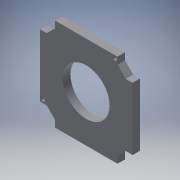
# Autodesk Inventor part: 20_Cube_Insert_CirAp_Guide
Saved by Autodesk Inventor 2019 (Build 230136000, 136)
## iProperties
Created: 2019-10-23
Part Number: 20_Cube_Insert_CirAp_Guide
Material: Generic
Document SubType Name: Modeling
Designer: marsikovabarbora
Density: 1 g/cm^3
Appearance: Default
Author: marsikovabarbora
Autodesk Inventor part; units mm, degrees
ref_plane "YZ Plane" through (0, 0, 0) normal (1, 0, 0) x (0, 1, 0)
ref_plane "XZ Plane" through (0, 0, 0) normal (0, 1, 0) x (-1, 0, 0)
ref_plane "XY Plane" through (0, 0, 0) normal (0, 0, 1) x (1, 0, 0)
sketch "Sketch1" plane through (0, 0, 0) normal (0, 0, 1) x (1, 0, 0)
  line L0 (-34.8609, 0) -> (34.8609, 0) construction
  line L1 (0, -34.8609) -> (0, 34.8609) construction
  line L2 (0, 0) -> (11.6542, 11.6542) construction
  line L3 (0, 0) -> (16.4815, 0) construction
  line L4 (0, 24.9006) -> (16.8, 24.9006)
  line L5 (16.8, 24.9006) -> (16.8, 21.2406)
  line L6 (16.8, 21.2406) -> (19.0203, 19.0203)
  line L7 (24.9006, 0) -> (24.9006, 16.8)
  line L8 (24.9006, 16.8) -> (21.2406, 16.8)
  line L9 (21.2406, 16.8) -> (19.0203, 19.0203)
  line L10 (0, 0) -> (-11.6542, 11.6542) construction
  line L11 (0, 0) -> (-16.4815, 0) construction
  line L12 (0, 24.9006) -> (-16.8, 24.9006)
  line L13 (-16.8, 24.9006) -> (-16.8, 21.2406)
  line L14 (-16.8, 21.2406) -> (-19.0203, 19.0203)
  line L15 (-24.9006, 0) -> (-24.9006, 16.8)
  line L16 (-24.9006, 16.8) -> (-21.2406, 16.8)
  line L17 (-21.2406, 16.8) -> (-19.0203, 19.0203)
  line L18 (0, 0) -> (11.6542, -11.6542) construction
  line L19 (0, -24.9006) -> (16.8, -24.9006)
  line L20 (16.8, -24.9006) -> (16.8, -21.2406)
  line L21 (16.8, -21.2406) -> (19.0203, -19.0203)
  line L22 (24.9006, 0) -> (24.9006, -16.8)
  line L23 (24.9006, -16.8) -> (21.2406, -16.8)
  line L24 (21.2406, -16.8) -> (19.0203, -19.0203)
  line L25 (0, 0) -> (-11.6542, -11.6542) construction
  line L26 (0, -24.9006) -> (-16.8, -24.9006)
  line L27 (-16.8, -24.9006) -> (-16.8, -21.2406)
  line L28 (-16.8, -21.2406) -> (-19.0203, -19.0203)
  line L29 (-24.9006, 0) -> (-24.9006, -16.8)
  line L30 (-24.9006, -16.8) -> (-21.2406, -16.8)
  line L31 (-21.2406, -16.8) -> (-19.0203, -19.0203)
  dimension "d0" = 45
  dimension "d1" = 3.14
  dimension "d2" = 3.66
  dimension "d3" = 16.8
  constraints: 60 end point, 24 symmetric about line, 5 point on line, 2 horizontal, 2 perpendicular, 1 equal length
  measures "d0" angle of L3 L2
  measures "d1" distance of L5.end L6.end
  measures "d2" distance of L4.end L5.end
  measures "d3" distance of L4.start L4.end
extrude "Extrusion1" add sketch "Sketch1" along normal blind 4
hole "Hole1" at (0, 0, 0) direction (0, 0, 1) diameter 26.6 end through all
sketch "Sketch6" plane through (0, 0, 4) normal (0, 0, 1) x (1, 0, 0)
  circle A0 centre (0, 0) radius 13.3 construction
  line L0 (16.8, 24.9006) -> (-16.8, 24.9006) construction
  line L1 (-16.8, 24.9006) -> (-16.8, 21.2406) construction
  line L2 (-16.8, 21.2406) -> (-21.2406, 16.8) construction
  line L3 (-21.2406, 16.8) -> (-24.9006, 16.8) construction
  line L4 (-24.9006, 16.8) -> (-24.9006, -16.8) construction
  line L5 (-24.9006, -16.8) -> (-21.2406, -16.8) construction
  line L6 (-21.2406, -16.8) -> (-16.8, -21.2406) construction
  line L7 (-16.8, -21.2406) -> (-16.8, -24.9006) construction
  line L8 (-16.8, -24.9006) -> (16.8, -24.9006) construction
  line L9 (16.8, -24.9006) -> (16.8, -21.2406) construction
  line L10 (16.8, -21.2406) -> (21.2406, -16.8) construction
  line L11 (21.2406, -16.8) -> (24.9006, -16.8) construction
  line L12 (24.9006, -16.8) -> (24.9006, 16.8) construction
  line L13 (24.9006, 16.8) -> (21.2406, 16.8) construction
  line L14 (21.2406, 16.8) -> (16.8, 21.2406) construction
  line L15 (16.8, 21.2406) -> (16.8, 24.9006) construction
  circle A1 centre (0, 0) radius 13.3
  circle A2 centre (0, 0) radius 13.5
  dimension "d42" = 26.6
  dimension "d43" = 27
  constraints: 2 centre point, 1 coincident, 1 concentric
  measures "d42" diameter of A1
  measures "d43" diameter of A2
extrude "Extrusion4" [suppressed]
sketch "Sketch7" plane through (0, 0, 0) normal (0, 0, -1) x (-1, 0, 0)
  line L0 (16.8, 24.9006) -> (-16.8, 24.9006) construction
  line L1 (-16.8, 24.9006) -> (-16.8, 21.2406) construction
  line L2 (-16.8, 21.2406) -> (-21.2406, 16.8) construction
  line L3 (-21.2406, 16.8) -> (-24.9006, 16.8) construction
  line L4 (-24.9006, 16.8) -> (-24.9006, -16.8) construction
  line L5 (-24.9006, -16.8) -> (-21.2406, -16.8) construction
  line L6 (-21.2406, -16.8) -> (-16.8, -21.2406) construction
  line L7 (-16.8, -21.2406) -> (-16.8, -24.9006) construction
  line L8 (-16.8, -24.9006) -> (16.8, -24.9006) construction
  line L9 (16.8, -24.9006) -> (16.8, -21.2406) construction
  line L10 (16.8, -21.2406) -> (21.2406, -16.8) construction
  line L11 (21.2406, -16.8) -> (24.9006, -16.8) construction
  line L12 (24.9006, -16.8) -> (24.9006, 16.8) construction
  line L13 (24.9006, 16.8) -> (21.2406, 16.8) construction
  line L14 (21.2406, 16.8) -> (16.8, 21.2406) construction
  line L15 (16.8, 21.2406) -> (16.8, 24.9006) construction
  line L16 (-2.0147, 24.1761) -> (-2, 24) construction
  line L17 (-1.9775, 24.0019) -> (-1.9921, 24.178) construction
  line L18 (1.9921, 24.178) -> (1.9775, 24.0019) construction
  line L19 (2, 24) -> (2.0147, 24.1761) construction
  line L20 (5.9445, 23.5204) -> (5.9012, 23.349) construction
  line L21 (5.923, 23.3435) -> (5.9665, 23.5148) construction
  line L22 (9.7347, 22.2212) -> (9.6638, 22.0593) construction
  line L23 (9.6844, 22.0502) -> (9.7555, 22.212) construction
  line L24 (13.2594, 20.3158) -> (13.1628, 20.1678) construction
  line L25 (13.1817, 20.1555) -> (13.2784, 20.3034) construction
  line L26 (16.4225, 17.8563) -> (16.3028, 17.7262) construction
  line L27 (16.3194, 17.7109) -> (16.4392, 17.8409) construction
  line L28 (19.1375, 14.9097) -> (18.9981, 14.8011) construction
  line L29 (19.0119, 14.7833) -> (19.1515, 14.8918) construction
  line L30 (21.3306, 11.5564) -> (21.1752, 11.4722) construction
  line L31 (21.1859, 11.4524) -> (21.3414, 11.5365) construction
  line L32 (22.9418, 7.8879) -> (22.7746, 7.8305) construction
  line L33 (22.782, 7.8091) -> (22.9492, 7.8665) construction
  line L34 (23.9272, 4.0042) -> (23.7529, 3.9751) construction
  line L35 (23.7566, 3.9529) -> (23.9309, 3.9819) construction
  line L36 (24.2599, 0.0113) -> (24.0832, 0.0113) construction
  line L37 (24.0832, -0.0113) -> (24.2599, -0.0113) construction
  line L38 (23.9309, -3.9819) -> (23.7566, -3.9529) construction
  line L39 (23.7529, -3.9751) -> (23.9272, -4.0042) construction
  line L40 (22.9492, -7.8665) -> (22.782, -7.8091) construction
  line L41 (22.7746, -7.8305) -> (22.9418, -7.8879) construction
  line L42 (21.3414, -11.5365) -> (21.1859, -11.4524) construction
  line L43 (21.1752, -11.4722) -> (21.3306, -11.5564) construction
  line L44 (19.1515, -14.8918) -> (19.0119, -14.7833) construction
  line L45 (18.9981, -14.8011) -> (19.1375, -14.9097) construction
  line L46 (16.4392, -17.8409) -> (16.3194, -17.7109) construction
  line L47 (16.3028, -17.7262) -> (16.4225, -17.8563) construction
  line L48 (13.2784, -20.3034) -> (13.1817, -20.1555) construction
  line L49 (13.1628, -20.1678) -> (13.2594, -20.3158) construction
  line L50 (9.7555, -22.212) -> (9.6844, -22.0502) construction
  line L51 (9.6638, -22.0593) -> (9.7347, -22.2212) construction
  line L52 (5.9665, -23.5148) -> (5.923, -23.3435) construction
  line L53 (5.9012, -23.349) -> (5.9445, -23.5204) construction
  line L54 (2.0147, -24.1761) -> (2, -24) construction
  line L55 (1.9775, -24.0019) -> (1.9921, -24.178) construction
  line L56 (-1.9921, -24.178) -> (-1.9775, -24.0019) construction
  line L57 (-2, -24) -> (-2.0147, -24.1761) construction
  line L58 (-5.9445, -23.5204) -> (-5.9012, -23.349) construction
  line L59 (-5.923, -23.3435) -> (-5.9665, -23.5148) construction
  line L60 (-9.7347, -22.2212) -> (-9.6638, -22.0593) construction
  line L61 (-9.6844, -22.0502) -> (-9.7555, -22.212) construction
  line L62 (-13.2594, -20.3158) -> (-13.1628, -20.1678) construction
  line L63 (-13.1817, -20.1555) -> (-13.2784, -20.3034) construction
  line L64 (-16.4225, -17.8563) -> (-16.3028, -17.7262) construction
  line L65 (-16.3194, -17.7109) -> (-16.4392, -17.8409) construction
  line L66 (-19.1375, -14.9097) -> (-18.9981, -14.8011) construction
  line L67 (-19.0119, -14.7833) -> (-19.1515, -14.8918) construction
  line L68 (-21.3306, -11.5564) -> (-21.1752, -11.4722) construction
  line L69 (-21.1859, -11.4524) -> (-21.3414, -11.5365) construction
  line L70 (-22.9418, -7.8879) -> (-22.7746, -7.8305) construction
  line L71 (-22.782, -7.8091) -> (-22.9492, -7.8665) construction
  line L72 (-23.9272, -4.0042) -> (-23.7529, -3.9751) construction
  line L73 (-23.7566, -3.9529) -> (-23.9309, -3.9819) construction
  line L74 (-24.2599, -0.0113) -> (-24.0832, -0.0113) construction
  line L75 (-24.0832, 0.0113) -> (-24.2599, 0.0113) construction
  line L76 (-23.9309, 3.9819) -> (-23.7566, 3.9529) construction
  line L77 (-23.7529, 3.9751) -> (-23.9272, 4.0042) construction
  line L78 (-22.9492, 7.8665) -> (-22.782, 7.8091) construction
  line L79 (-22.7746, 7.8305) -> (-22.9418, 7.8879) construction
  line L80 (-21.3414, 11.5365) -> (-21.1859, 11.4524) construction
  line L81 (-21.1752, 11.4722) -> (-21.3306, 11.5564) construction
  line L82 (-19.1515, 14.8918) -> (-19.0119, 14.7833) construction
  line L83 (-18.9981, 14.8011) -> (-19.1375, 14.9097) construction
  line L84 (-16.4392, 17.8409) -> (-16.3194, 17.7109) construction
  line L85 (-16.3028, 17.7262) -> (-16.4225, 17.8563) construction
  line L86 (-13.2784, 20.3034) -> (-13.1817, 20.1555) construction
  line L87 (-13.1628, 20.1678) -> (-13.2594, 20.3158) construction
  line L88 (-9.7555, 22.212) -> (-9.6844, 22.0502) construction
  line L89 (-9.6638, 22.0593) -> (-9.7347, 22.2212) construction
  line L90 (-5.9665, 23.5148) -> (-5.923, 23.3435) construction
  line L91 (-5.9012, 23.349) -> (-5.9445, 23.5204) construction
  circle A0 centre (0, 24.5946) radius 2 construction
  line L92 (2, 33.2113) -> (-2, 33.2113)
  line L93 (-2, 33.2113) -> (-2, 6.8481)
  line L94 (-2, 6.8481) -> (2, 6.8481)
  line L95 (2, 6.8481) -> (2, 33.2113)
  circle A1 centre (-17.7867, 14.1844) radius 1.25 projected
  circle A2 centre (-22.1796, -5.0624) radius 1.25 projected
  circle A3 centre (-9.8709, -20.497) radius 1.25 projected
  circle A4 centre (9.8709, -20.497) radius 1.25 projected
  circle A5 centre (22.1796, -5.0624) radius 1.25 projected
  circle A6 centre (17.7867, 14.1844) radius 1.25 projected
  circle A7 centre (0, 22.75) radius 1.25 projected
  arc A8 (-2.0147, 24.1761) -> (-5.9445, 23.5204) centre (-3.9503, 23.6727) ccw projected
  arc A9 (-1.9973, 24.1039) -> (-2, 24) centre (0, 24) ccw projected
  arc A10 (-1.9775, 24.0019) -> (-1.9973, 24.1039) centre (-3.9503, 23.6727) ccw projected
  arc A11 (1.9921, 24.178) -> (-1.9921, 24.178) centre (0, 24) ccw projected
  arc A12 (1.9973, 24.1039) -> (1.9775, 24.0019) centre (3.9503, 23.6727) ccw projected
  arc A13 (2, 24) -> (1.9973, 24.1039) centre (0, 24) ccw projected
  arc A14 (5.9445, 23.5204) -> (2.0147, 24.1761) centre (3.9503, 23.6727) ccw projected
  arc A15 (5.9374, 23.4464) -> (5.9012, 23.349) centre (7.7928, 22.6996) ccw projected
  arc A16 (5.923, 23.3435) -> (5.9374, 23.4464) centre (3.9503, 23.6727) ccw projected
  arc A17 (9.7347, 22.2212) -> (5.9665, 23.5148) centre (7.7928, 22.6996) ccw projected
  arc A18 (9.7156, 22.1493) -> (9.6638, 22.0593) centre (11.4227, 21.1074) ccw projected
  arc A19 (9.6844, 22.0502) -> (9.7156, 22.1493) centre (7.7928, 22.6996) ccw projected
  arc A20 (13.2594, 20.3158) -> (9.7555, 22.212) centre (11.4227, 21.1074) ccw projected
  arc A21 (13.2287, 20.2481) -> (13.1628, 20.1678) centre (14.7411, 18.9394) ccw projected
  arc A22 (13.1817, 20.1555) -> (13.2287, 20.2481) centre (11.4227, 21.1074) ccw projected
  arc A23 (16.4225, 17.8563) -> (13.2784, 20.3034) centre (14.7411, 18.9394) ccw projected
  arc A24 (16.381, 17.7946) -> (16.3028, 17.7262) centre (17.6574, 16.2548) ccw projected
  arc A25 (16.3194, 17.7109) -> (16.381, 17.7946) centre (14.7411, 18.9394) ccw projected
  arc A26 (19.1375, 14.9097) -> (16.4392, 17.8409) centre (17.6574, 16.2548) ccw projected
  arc A27 (19.0865, 14.8556) -> (18.9981, 14.8011) centre (20.092, 13.1268) ccw projected
  arc A28 (19.0119, 14.7833) -> (19.0865, 14.8556) centre (17.6574, 16.2548) ccw projected
  arc A29 (21.3306, 11.5564) -> (19.1515, 14.8918) centre (20.092, 13.1268) ccw projected
  arc A30 (21.2714, 11.5115) -> (21.1752, 11.4722) centre (21.9786, 9.6407) ccw projected
  arc A31 (21.1859, 11.4524) -> (21.2714, 11.5115) centre (20.092, 13.1268) ccw projected
  arc A32 (22.9418, 7.8879) -> (21.3414, 11.5365) centre (21.9786, 9.6407) ccw projected
  arc A33 (22.876, 7.8533) -> (22.7746, 7.8305) centre (23.2656, 5.8917) ccw projected
  arc A34 (22.782, 7.8091) -> (22.876, 7.8533) centre (21.9786, 9.6407) ccw projected
  arc A35 (23.9272, 4.0042) -> (22.9492, 7.8665) centre (23.2656, 5.8917) ccw projected
  arc A36 (23.8566, 3.981) -> (23.7529, 3.9751) centre (23.918, 1.9819) ccw projected
  arc A37 (23.7566, 3.9529) -> (23.8566, 3.981) centre (23.2656, 5.8917) ccw projected
  arc A38 (24.2599, 0.0113) -> (23.9309, 3.9819) centre (23.918, 1.9819) ccw projected
  arc A39 (24.1865, 0) -> (24.0832, 0.0113) centre (23.918, -1.9819) ccw projected
  arc A40 (24.0832, -0.0113) -> (24.1865, 0) centre (23.918, 1.9819) ccw projected
  arc A41 (23.9309, -3.9819) -> (24.2599, -0.0113) centre (23.918, -1.9819) ccw projected
  arc A42 (23.8566, -3.981) -> (23.7566, -3.9529) centre (23.2656, -5.8917) ccw projected
  arc A43 (23.7529, -3.9751) -> (23.8566, -3.981) centre (23.918, -1.9819) ccw projected
  arc A44 (22.9492, -7.8665) -> (23.9272, -4.0042) centre (23.2656, -5.8917) ccw projected
  arc A45 (22.876, -7.8533) -> (22.782, -7.8091) centre (21.9786, -9.6407) ccw projected
  arc A46 (22.7746, -7.8305) -> (22.876, -7.8533) centre (23.2656, -5.8917) ccw projected
  arc A47 (21.3414, -11.5365) -> (22.9418, -7.8879) centre (21.9786, -9.6407) ccw projected
  arc A48 (21.2714, -11.5115) -> (21.1859, -11.4524) centre (20.092, -13.1268) ccw projected
  arc A49 (21.1752, -11.4722) -> (21.2714, -11.5115) centre (21.9786, -9.6407) ccw projected
  arc A50 (19.1515, -14.8918) -> (21.3306, -11.5564) centre (20.092, -13.1268) ccw projected
  arc A51 (19.0865, -14.8556) -> (19.0119, -14.7833) centre (17.6574, -16.2548) ccw projected
  arc A52 (18.9981, -14.8011) -> (19.0865, -14.8556) centre (20.092, -13.1268) ccw projected
  arc A53 (16.4392, -17.8409) -> (19.1375, -14.9097) centre (17.6574, -16.2548) ccw projected
  arc A54 (16.381, -17.7946) -> (16.3194, -17.7109) centre (14.7411, -18.9394) ccw projected
  arc A55 (16.3028, -17.7262) -> (16.381, -17.7946) centre (17.6574, -16.2548) ccw projected
  arc A56 (13.2784, -20.3034) -> (16.4225, -17.8563) centre (14.7411, -18.9394) ccw projected
  arc A57 (13.2287, -20.2481) -> (13.1817, -20.1555) centre (11.4227, -21.1074) ccw projected
  arc A58 (13.1628, -20.1678) -> (13.2287, -20.2481) centre (14.7411, -18.9394) ccw projected
  arc A59 (9.7555, -22.212) -> (13.2594, -20.3158) centre (11.4227, -21.1074) ccw projected
  arc A60 (9.7156, -22.1493) -> (9.6844, -22.0502) centre (7.7928, -22.6996) ccw projected
  arc A61 (9.6638, -22.0593) -> (9.7156, -22.1493) centre (11.4227, -21.1074) ccw projected
  arc A62 (5.9665, -23.5148) -> (9.7347, -22.2212) centre (7.7928, -22.6996) ccw projected
  arc A63 (5.9374, -23.4464) -> (5.923, -23.3435) centre (3.9503, -23.6727) ccw projected
  arc A64 (5.9012, -23.349) -> (5.9374, -23.4464) centre (7.7928, -22.6996) ccw projected
  arc A65 (2.0147, -24.1761) -> (5.9445, -23.5204) centre (3.9503, -23.6727) ccw projected
  arc A66 (1.9973, -24.1039) -> (2, -24) centre (0, -24) ccw projected
  arc A67 (1.9775, -24.0019) -> (1.9973, -24.1039) centre (3.9503, -23.6727) ccw projected
  arc A68 (-1.9921, -24.178) -> (1.9921, -24.178) centre (0, -24) ccw projected
  arc A69 (-1.9973, -24.1039) -> (-1.9775, -24.0019) centre (-3.9503, -23.6727) ccw projected
  arc A70 (-2, -24) -> (-1.9973, -24.1039) centre (0, -24) ccw projected
  arc A71 (-5.9445, -23.5204) -> (-2.0147, -24.1761) centre (-3.9503, -23.6727) ccw projected
  arc A72 (-5.9374, -23.4464) -> (-5.9012, -23.349) centre (-7.7928, -22.6996) ccw projected
  arc A73 (-5.923, -23.3435) -> (-5.9374, -23.4464) centre (-3.9503, -23.6727) ccw projected
  arc A74 (-9.7347, -22.2212) -> (-5.9665, -23.5148) centre (-7.7928, -22.6996) ccw projected
  arc A75 (-9.7156, -22.1493) -> (-9.6638, -22.0593) centre (-11.4227, -21.1074) ccw projected
  arc A76 (-9.6844, -22.0502) -> (-9.7156, -22.1493) centre (-7.7928, -22.6996) ccw projected
  arc A77 (-13.2594, -20.3158) -> (-9.7555, -22.212) centre (-11.4227, -21.1074) ccw projected
  arc A78 (-13.2287, -20.2481) -> (-13.1628, -20.1678) centre (-14.7411, -18.9394) ccw projected
  arc A79 (-13.1817, -20.1555) -> (-13.2287, -20.2481) centre (-11.4227, -21.1074) ccw projected
  arc A80 (-16.4225, -17.8563) -> (-13.2784, -20.3034) centre (-14.7411, -18.9394) ccw projected
  arc A81 (-16.381, -17.7946) -> (-16.3028, -17.7262) centre (-17.6574, -16.2548) ccw projected
  arc A82 (-16.3194, -17.7109) -> (-16.381, -17.7946) centre (-14.7411, -18.9394) ccw projected
  arc A83 (-19.1375, -14.9097) -> (-16.4392, -17.8409) centre (-17.6574, -16.2548) ccw projected
  arc A84 (-19.0865, -14.8556) -> (-18.9981, -14.8011) centre (-20.092, -13.1268) ccw projected
  arc A85 (-19.0119, -14.7833) -> (-19.0865, -14.8556) centre (-17.6574, -16.2548) ccw projected
  arc A86 (-21.3306, -11.5564) -> (-19.1515, -14.8918) centre (-20.092, -13.1268) ccw projected
  arc A87 (-21.2714, -11.5115) -> (-21.1752, -11.4722) centre (-21.9786, -9.6407) ccw projected
  arc A88 (-21.1859, -11.4524) -> (-21.2714, -11.5115) centre (-20.092, -13.1268) ccw projected
  arc A89 (-22.9418, -7.8879) -> (-21.3414, -11.5365) centre (-21.9786, -9.6407) ccw projected
  arc A90 (-22.876, -7.8533) -> (-22.7746, -7.8305) centre (-23.2656, -5.8917) ccw projected
  arc A91 (-22.782, -7.8091) -> (-22.876, -7.8533) centre (-21.9786, -9.6407) ccw projected
  arc A92 (-23.9272, -4.0042) -> (-22.9492, -7.8665) centre (-23.2656, -5.8917) ccw projected
  arc A93 (-23.8566, -3.981) -> (-23.7529, -3.9751) centre (-23.918, -1.9819) ccw projected
  arc A94 (-23.7566, -3.9529) -> (-23.8566, -3.981) centre (-23.2656, -5.8917) ccw projected
  arc A95 (-24.2599, -0.0113) -> (-23.9309, -3.9819) centre (-23.918, -1.9819) ccw projected
  arc A96 (-24.1865, 0) -> (-24.0832, -0.0113) centre (-23.918, 1.9819) ccw projected
  arc A97 (-24.0832, 0.0113) -> (-24.1865, 0) centre (-23.918, -1.9819) ccw projected
  arc A98 (-23.9309, 3.9819) -> (-24.2599, 0.0113) centre (-23.918, 1.9819) ccw projected
  arc A99 (-23.8566, 3.981) -> (-23.7566, 3.9529) centre (-23.2656, 5.8917) ccw projected
  arc A100 (-23.7529, 3.9751) -> (-23.8566, 3.981) centre (-23.918, 1.9819) ccw projected
  arc A101 (-22.9492, 7.8665) -> (-23.9272, 4.0042) centre (-23.2656, 5.8917) ccw projected
  arc A102 (-22.876, 7.8533) -> (-22.782, 7.8091) centre (-21.9786, 9.6407) ccw projected
  arc A103 (-22.7746, 7.8305) -> (-22.876, 7.8533) centre (-23.2656, 5.8917) ccw projected
  arc A104 (-21.3414, 11.5365) -> (-22.9418, 7.8879) centre (-21.9786, 9.6407) ccw projected
  arc A105 (-21.2714, 11.5115) -> (-21.1859, 11.4524) centre (-20.092, 13.1268) ccw projected
  arc A106 (-21.1752, 11.4722) -> (-21.2714, 11.5115) centre (-21.9786, 9.6407) ccw projected
  arc A107 (-19.1515, 14.8918) -> (-21.3306, 11.5564) centre (-20.092, 13.1268) ccw projected
  arc A108 (-19.0865, 14.8556) -> (-19.0119, 14.7833) centre (-17.6574, 16.2548) ccw projected
  arc A109 (-18.9981, 14.8011) -> (-19.0865, 14.8556) centre (-20.092, 13.1268) ccw projected
  arc A110 (-16.4392, 17.8409) -> (-19.1375, 14.9097) centre (-17.6574, 16.2548) ccw projected
  arc A111 (-16.381, 17.7946) -> (-16.3194, 17.7109) centre (-14.7411, 18.9394) ccw projected
  arc A112 (-16.3028, 17.7262) -> (-16.381, 17.7946) centre (-17.6574, 16.2548) ccw projected
  arc A113 (-13.2784, 20.3034) -> (-16.4225, 17.8563) centre (-14.7411, 18.9394) ccw projected
  arc A114 (-13.2287, 20.2481) -> (-13.1817, 20.1555) centre (-11.4227, 21.1074) ccw projected
  arc A115 (-13.1628, 20.1678) -> (-13.2287, 20.2481) centre (-14.7411, 18.9394) ccw projected
  arc A116 (-9.7555, 22.212) -> (-13.2594, 20.3158) centre (-11.4227, 21.1074) ccw projected
  arc A117 (-9.7156, 22.1493) -> (-9.6844, 22.0502) centre (-7.7928, 22.6996) ccw projected
  arc A118 (-9.6638, 22.0593) -> (-9.7156, 22.1493) centre (-11.4227, 21.1074) ccw projected
  arc A119 (-5.9665, 23.5148) -> (-9.7347, 22.2212) centre (-7.7928, 22.6996) ccw projected
  arc A120 (-5.9374, 23.4464) -> (-5.923, 23.3435) centre (-3.9503, 23.6727) ccw projected
  arc A121 (-5.9012, 23.349) -> (-5.9374, 23.4464) centre (-7.7928, 22.6996) ccw projected
  circle A122 centre (0, 0) radius 21 projected
  point P0 (0, 0)
  point P1 (3.35, 15.4344)
  point P2 (3.35, -6.3124)
  point P3 (3.35, 24.1039)
  point P4 (3.35, 24.1039)
  point P5 (3.35, 25.6727)
  point P6 (3.35, 23.4464)
  point P7 (3.35, 20.3158)
  point P8 (3.35, 20.2481)
  point P9 (3.35, 17.7946)
  point P10 (3.35, 14.8556)
  point P11 (3.35, 11.5115)
  point P12 (3.35, 7.8533)
  point P13 (3.35, 3.981)
  point P14 (3.35, 0.0113)
  point P15 (3.35, 0)
  point P16 (3.35, -3.981)
  point P17 (3.35, -7.8533)
  point P18 (3.35, -11.5115)
  point P19 (3.35, -14.8556)
  point P20 (3.35, -18.2548)
  point P21 (3.35, -17.7946)
  point P22 (3.35, -20.2481)
  point P23 (3.35, -22.1493)
  point P24 (3.35, -23.4464)
  point P25 (3.35, -24.1039)
  point P26 (3.35, -24.1039)
  point P27 (3.35, -25.6727)
  point P28 (3.35, -23.4464)
  point P29 (3.35, -20.3158)
  point P30 (3.35, -20.1555)
  point P31 (3.35, -17.7109)
  point P32 (3.35, -14.7833)
  point P33 (3.35, -11.4524)
  point P34 (3.35, -7.8091)
  point P35 (3.35, -3.9529)
  point P36 (3.35, -0.0113)
  point P37 (3.35, 0.0113)
  point P38 (3.35, 3.981)
  point P39 (3.35, 7.8533)
  point P40 (3.35, 11.5115)
  point P41 (3.35, 14.8556)
  point P42 (3.35, 18.2548)
  point P43 (3.35, 17.7946)
  point P44 (3.35, 20.2481)
  point P45 (3.35, 22.1493)
  point P46 (3.35, 23.4464)
  dimension "d32" = 4
  constraints: 8 end point, 2 parallel, 2 tangent, 1 centre point, 1 horizontal, 1 perpendicular, 38 other
  measures "d32" diameter of A0
extrude "Extrusion5" cut sketch "Sketch7" against normal blind 2 contours L95 A122 L93 L92 | L95 L94 L93 A122 | A7 picked at (0.2225, 11.5619)
pattern_circular "Circular Pattern1" count 7 over 360 about axis through (0, 0, -10) along (0, 0, 1) of "Extrusion5"
sketch "Sketch8" plane through (0, 0, 4) normal (0, 0, 1) x (1, 0, 0)
  line L0 (16.8, 24.9006) -> (-16.8, 24.9006) projected
  line L1 (-16.8, 24.9006) -> (-16.8, 21.2406) projected
  line L2 (-16.8, 21.2406) -> (-21.2406, 16.8) projected
  line L3 (-21.2406, 16.8) -> (-24.9006, 16.8) projected
  line L4 (-24.9006, 16.8) -> (-24.9006, -16.8) projected
  line L5 (-24.9006, -16.8) -> (-21.2406, -16.8) projected
  line L6 (-21.2406, -16.8) -> (-16.8, -21.2406) projected
  line L7 (-16.8, -21.2406) -> (-16.8, -24.9006) projected
  line L8 (-16.8, -24.9006) -> (16.8, -24.9006) projected
  line L9 (16.8, -24.9006) -> (16.8, -21.2406) projected
  line L10 (16.8, -21.2406) -> (21.2406, -16.8) projected
  line L11 (21.2406, -16.8) -> (24.9006, -16.8) projected
  line L12 (24.9006, -16.8) -> (24.9006, 16.8) projected
  line L13 (24.9006, 16.8) -> (21.2406, 16.8) projected
  line L14 (21.2406, 16.8) -> (16.8, 21.2406) projected
  line L15 (16.8, 21.2406) -> (16.8, 24.9006) projected
  line L16 (-23.9006, -15.8) -> (-23.9006, 15.8)
  line L17 (-23.9006, 15.8) -> (-20.8264, 15.8)
  line L18 (-20.8264, 15.8) -> (-15.8, 20.8264)
  line L19 (-15.8, 20.8264) -> (-15.8, 23.9006)
  line L20 (-15.8, 23.9006) -> (15.8, 23.9006)
  line L21 (15.8, 23.9006) -> (15.8, 20.8264)
  line L22 (15.8, 20.8264) -> (20.8264, 15.8)
  line L23 (20.8264, 15.8) -> (23.9006, 15.8)
  line L24 (23.9006, 15.8) -> (23.9006, -15.8)
  line L25 (23.9006, -15.8) -> (20.8264, -15.8)
  line L26 (20.8264, -15.8) -> (15.8, -20.8264)
  line L27 (15.8, -20.8264) -> (15.8, -23.9006)
  line L28 (15.8, -23.9006) -> (-15.8, -23.9006)
  line L29 (-15.8, -23.9006) -> (-15.8, -20.8264)
  line L30 (-15.8, -20.8264) -> (-20.8264, -15.8)
  line L31 (-20.8264, -15.8) -> (-23.9006, -15.8)
  circle A0 centre (0, 0) radius 13.3 projected
  circle A1 centre (0, 0) radius 12.5
  dimension "d41" = 1
  dimension "d46" = 0.8
  constraints: 32 end point, 1 centre point, 15 other
  measures "d41" distance between parallel lines of L4 L16
  measures "d46" radial gap between concentric circles of A0 A1
extrude "Extrusion6" add sketch "Sketch8" against normal up to surface (4 mm away)
sketch "Sketch9" plane through (0, 0, 0) normal (0, 0, -1) x (-1, 0, 0)
  circle A0 centre (-23.1006, 15) radius 1.05 projected
  circle A1 centre (23.1006, -15) radius 1.05 projected
  point P0 (0, 0)
extrude "Extrusion7" cut sketch "Sketch9" against normal through all
body "Solid1"
